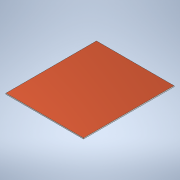
# Autodesk Inventor part: Baquelita
Saved by Autodesk Inventor 2020 (Build 240168000, 168)
## iProperties
Created: 2021-10-19
Part Number: Baquelita
Material: Genérico
Document SubType Name: Modeling
Designer: DANIEL
Density: 1 g/cm^3
Appearance: Valor por defecto
Author: DANIEL
Autodesk Inventor part; units mm, degrees
ref_plane "YZ Plane" through (0, 0, 0) normal (1, 0, 0) x (0, 1, 0)
ref_plane "XZ Plane" through (0, 0, 0) normal (0, 1, 0) x (-1, 0, 0)
ref_plane "XY Plane" through (0, 0, 0) normal (0, 0, 1) x (1, 0, 0)
sketch "Boceto1" plane through (0, 0, 0) normal (0, 1, 0) x (-1, 0, 0)
  line L0 (39, 45.5) -> (-39, 45.5)
  line L1 (-39, 45.5) -> (-39, -45.5)
  line L2 (-39, -45.5) -> (39, -45.5)
  line L3 (39, -45.5) -> (39, 45.5)
  point P0 (0, 0)
  dimension "w" = 91
  dimension "d3" = 45.5
  dimension "k" = 78
  dimension "d7" = 39
  constraints: 8 end point, 2 parallel, 1 horizontal, 1 perpendicular
  measures "w" distance between parallel lines of L2 L0
  measures "d3" distance from line of L0 point (0, 0)
  measures "k" distance between parallel lines of L1 L3
  measures "d7" distance from line of L3 point (0, 0)
extrude "Extrusión1" add sketch "Boceto1" along normal blind 1
equation "\"d3\" = 0.5 * w"
equation "\"d7\" = 0.5 * k"
